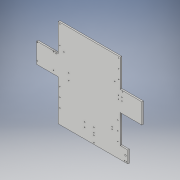
# Autodesk Inventor part: Gen2PlatePart
Saved by Autodesk Inventor 2019 (Build 230136000, 136)
## iProperties
Created: 2017-12-06
Part Number: Gen2PlatePart
Material: Generic
Document SubType Name: Modeling
Designer: User
Density: 1 g/cm^3
Appearance: Default
Mass: 688.034 g
Surface Area: 2294.14 cm^2
Volume: 688.034 cm^3
Author: User
Autodesk Inventor part; units mm, degrees
ref_plane "YZ Plane" through (0, 0, 0) normal (1, 0, 0) x (0, 1, 0)
ref_plane "XZ Plane" through (0, 0, 0) normal (0, 1, 0) x (-1, 0, 0)
ref_plane "XY Plane" through (0, 0, 0) normal (0, 0, 1) x (1, 0, 0)
ref_plane "Work Plane32" through (254, 330.2, 0) normal (0, 0, -1) x (-1, 0, 0)
sketch "Sketch36" plane through (254, 330.2, 0) normal (0, 0, -1) x (-1, 0, 0)
  line L0 (254, -363.855) -> (254, -196.85) projected
  line L1 (0, 0) -> (0, -114.3) projected
  line L2 (254, -363.855) -> (0, -363.855)
  line L3 (0, -363.855) -> (0, 0)
  line L4 (0, 0) -> (254, 0)
  line L5 (254, 0) -> (254, -363.855)
  line L6 (342.9, -196.85) -> (342.9, -114.3) projected
  line L7 (342.9, -196.85) -> (254, -196.85)
  line L8 (254, -196.85) -> (254, -114.3)
  line L9 (254, -114.3) -> (342.9, -114.3)
  line L10 (342.9, -114.3) -> (342.9, -196.85)
  line L11 (-31.75, -363.855) -> (254, -363.855) projected
  line L12 (0, -314.325) -> (0, -196.85) projected
  line L13 (-31.75, -363.855) -> (0, -363.855)
  line L14 (0, -363.855) -> (0, -314.325)
  line L15 (0, -314.325) -> (-31.75, -314.325)
  line L16 (-31.75, -314.325) -> (-31.75, -363.855)
  line L17 (0, -196.85) -> (-88.9, -196.85)
  line L18 (-88.9, -196.85) -> (-88.9, -114.3)
  line L19 (-88.9, -114.3) -> (0, -114.3)
  line L20 (0, -114.3) -> (0, -196.85)
  point P0 (254, -330.2)
  constraints: 32 end point, 8 parallel, 4 horizontal, 4 perpendicular, 1 point on line
extrude "Extrusion20" add sketch "Sketch36" along normal blind 6.35
ref_plane "Work Plane28" through (254, 330.2, -6.35) normal (0, 0, -1) x (-1, 0, 0)
sketch "Sketch38" plane through (254, 330.2, -6.35) normal (0, 0, -1) x (-1, 0, 0)
  circle A0 centre (247.65, -304.8) radius 1.651 projected
  circle A1 centre (247.65, -304.8) radius 1.651
  circle A2 centre (247.65, -266.7) radius 1.651 projected
  circle A3 centre (247.65, -266.7) radius 1.651
  circle A4 centre (247.65, -228.6) radius 1.651 projected
  circle A5 centre (247.65, -228.6) radius 1.651
  circle A6 centre (273.685, -183.515) radius 1.778 projected
  circle A7 centre (273.685, -183.515) radius 1.778
  circle A8 centre (339.725, -183.515) radius 1.778 projected
  circle A9 centre (339.725, -183.515) radius 1.778
  circle A10 centre (339.725, -117.475) radius 1.778 projected
  circle A11 centre (339.725, -117.475) radius 1.778
  circle A12 centre (273.685, -117.475) radius 1.778 projected
  circle A13 centre (273.685, -117.475) radius 1.778
  circle A14 centre (263.1059, -119.0625) radius 1.778 projected
  circle A15 centre (263.1059, -119.0625) radius 1.778
  circle A16 centre (231.3559, -97.4725) radius 1.778 projected
  circle A17 centre (231.3559, -97.4725) radius 1.778
  circle A18 centre (247.65, -82.55) radius 1.651 projected
  circle A19 centre (247.65, -82.55) radius 1.651
  circle A20 centre (247.65, -6.35) radius 1.651 projected
  circle A21 centre (247.65, -6.35) radius 1.651
  circle A22 centre (211.2772, -162.052) radius 1.778 projected
  circle A23 centre (211.2772, -162.052) radius 1.778
  circle A24 centre (211.2772, -189.0014) radius 1.778 projected
  circle A25 centre (211.2772, -189.0014) radius 1.778
  circle A26 centre (6.35, -6.35) radius 1.651 projected
  circle A27 centre (6.35, -6.35) radius 1.651
  circle A28 centre (6.35, -44.45) radius 1.651 projected
  circle A29 centre (6.35, -44.45) radius 1.651
  circle A30 centre (6.35, -82.55) radius 1.651 projected
  circle A31 centre (6.35, -82.55) radius 1.651
  circle A32 centre (22.6441, -97.4725) radius 1.778 projected
  circle A33 centre (22.6441, -97.4725) radius 1.778
  circle A34 centre (-9.1059, -119.0625) radius 1.778 projected
  circle A35 centre (-9.1059, -119.0625) radius 1.778
  circle A36 centre (-6.9148, -139.1352) radius 1.778 projected
  circle A37 centre (-6.9148, -139.1352) radius 1.778
  circle A38 centre (6.9148, -139.1352) radius 1.778 projected
  circle A39 centre (6.9148, -139.1352) radius 1.778
  circle A40 centre (6.9148, -152.9648) radius 1.778 projected
  circle A41 centre (6.9148, -152.9648) radius 1.778
  circle A42 centre (-6.9148, -152.9648) radius 1.778 projected
  circle A43 centre (-6.9148, -152.9648) radius 1.778
  circle A44 centre (10.1373, -228.6) radius 1.651 projected
  circle A45 centre (10.1373, -228.6) radius 1.651
  circle A46 centre (10.1373, -266.7) radius 1.651 projected
  circle A47 centre (10.1373, -266.7) radius 1.651
  circle A48 centre (10.1373, -304.8) radius 1.651 projected
  circle A49 centre (10.1373, -304.8) radius 1.651
  circle A50 centre (32.893, -264.0838) radius 1.778 projected
  circle A51 centre (32.893, -264.0838) radius 1.778
  circle A52 centre (32.893, -272.9738) radius 1.778 projected
  circle A53 centre (32.893, -272.9738) radius 1.778
  circle A54 centre (-21.75, -337.98) radius 3.3782 projected
  circle A55 centre (-21.75, -337.98) radius 3.3782
  circle A56 centre (-18.1, -358.648) radius 1.778 projected
  circle A57 centre (-18.1, -358.648) radius 1.778
  circle A58 centre (-25.4, -358.648) radius 1.778 projected
  circle A59 centre (-25.4, -358.648) radius 1.778
  circle A60 centre (107.95, -332.105) radius 1.905 projected
  circle A61 centre (107.95, -332.105) radius 1.905
  circle A62 centre (107.95, -322.58) radius 1.905 projected
  circle A63 centre (107.95, -322.58) radius 1.905
  circle A64 centre (107.95, -303.53) radius 1.905 projected
  circle A65 centre (107.95, -303.53) radius 1.905
  circle A66 centre (107.95, -357.505) radius 1.905 projected
  circle A67 centre (107.95, -357.505) radius 1.905
  circle A68 centre (146.05, -303.53) radius 1.905 projected
  circle A69 centre (146.05, -303.53) radius 1.905
  circle A70 centre (146.05, -322.58) radius 1.905 projected
  circle A71 centre (146.05, -322.58) radius 1.905
  point P0 (254, -330.2)
  constraints: 36 centre point, 36 coincident
extrude "Extrusion21" cut sketch "Sketch38" against normal blind 6.35
body "Solid1"
